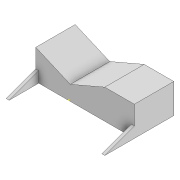
# Autodesk Inventor part: Modelo base
Saved by Autodesk Inventor 2022 (Build 260153000, 153)
## iProperties
Created: 2022-06-06
Part Number: Modelo base
Material: Generic
Document SubType Name: Modeling
Designer: ADMIN
Density: 1 g/cm^3
Appearance: Default
Author: ADMIN
Autodesk Inventor part; units mm, degrees
ref_plane "YZ Plane" through (0, 0, 0) normal (1, 0, 0) x (0, 1, 0)
ref_plane "XZ Plane" through (0, 0, 0) normal (0, 1, 0) x (-1, 0, 0)
ref_plane "XY Plane" through (0, 0, 0) normal (0, 0, 1) x (1, 0, 0)
sketch "Sketch1" plane through (0, 0, 0) normal (0, 0, 1) x (1, 0, 0)
  line L0 (-168.866, -3.5052) -> (-168.866, 146.4948)
  line L1 (-168.866, 146.4948) -> (6.134, 71.4948)
  line L2 (6.134, 71.4948) -> (181.134, 146.4948)
  line L3 (181.134, 146.4948) -> (181.134, -3.5052)
  line L4 (181.134, -3.5052) -> (-168.866, -3.5052)
  line L5 (181.134, 146.4948) -> (331.134, 146.4948)
  line L6 (331.134, 146.4948) -> (331.134, -3.5052)
  line L7 (331.134, -3.5052) -> (181.134, -3.5052)
  point P0 (0, 0)
  dimension "d0" = 350
  dimension "d1" = 150
  dimension "d2" = 150
  dimension "d3" = 175
  dimension "d4" = 75
  dimension "d5" = 150
  constraints: 16 end point, 3 perpendicular, 1 horizontal, 1 parallel, 1 vertical
  measures "d0" distance of L3.end L0.start
  measures "d1" distance of L0.start L0.end
  measures "d2" distance of L2.end L3.end
  measures "d3" horizontal distance of L0.end L1.end
  measures "d4" distance from line of L4 L1.end
  measures "d5" distance of L2.end L5.end
extrude "Extrusion1" add sketch "Sketch1" along normal blind 200
sketch "Sketch2" plane through (0, 0, 200) normal (0, 0, 1) x (1, 0, 0)
  point P0 (0, 0)
sketch "Sketch3" plane through (331.134, -3.5052, 0) normal (1, 0, 0) x (0, 0, -1)
  line L0 (0, 0) -> (0, 150) projected
  line L1 (0, 150) -> (-200, 150) projected
  line L2 (-200, 0) -> (-200, 150) projected
  line L3 (0, 0) -> (-200, 0) projected
  line L4 (-200, 0) -> (-350, 0)
  line L5 (-350, 0) -> (-200, 54.5955)
  line L6 (-200, 0) -> (-200, 150) projected
  point P0 (0, 3.5052)
  dimension "d12" = 20
  dimension "d13" = 150
  constraints: 4 end point, 1 horizontal, 1 point on line
  measures "d12" angle of L4 L5
  measures "d13" distance of L2.start L4.end
extrude "Extrusion2" add sketch "Sketch3" against normal blind 15 contours L4 L5 L2
sketch "Sketch4" plane through (-168.866, -3.5052, 0) normal (-1, 0, 0) x (0, 0, 1)
  line L0 (200, 0) -> (200, 54.5955) projected
  line L1 (200, 0) -> (350, 0) projected
  line L2 (350, 0) -> (200, 54.5955) projected
  point P0 (0, 3.5052)
extrude "Extrusion3" add sketch "Sketch4" against normal blind 15
equation "\"d2\" = d1"
equation "\"d3\" = 0.5 * d0"
body "Solid1"
